Autodesk Fusion 360 part; units mm, degrees
(part 2 of 4)
  line L389 (379.0066, 108.4473) -> (374.6816, 115.9384)
  line L390 (374.6816, 115.9384) -> (377.3663, 117.4884)
  line L391 (377.3663, 117.4884) -> (381.6913, 109.9973)
  line L392 (383.1913, 109.9973) -> (394.9765, 130.4099)
  line L393 (394.2265, 131.7089) -> (385.5765, 131.7089)
  line L394 (385.5765, 131.7089) -> (385.5765, 134.8089)
  line L395 (385.5765, 134.8089) -> (394.2265, 134.8089)
  line L396 (394.9765, 136.1079) -> (383.1913, 156.5205)
  line L397 (381.6913, 156.5205) -> (377.3663, 149.0294)
  line L398 (377.3663, 149.0294) -> (374.6816, 150.5794)
  line L399 (374.6816, 150.5794) -> (379.0066, 158.0705)
  line L400 (378.2566, 159.3696) -> (354.6862, 159.3696)
  line L401 (353.9362, 158.0705) -> (358.2612, 150.5794)
  line L402 (358.2612, 150.5794) -> (355.5765, 149.0294)
  line L403 (355.5765, 149.0294) -> (351.2515, 156.5205)
  line L404 (349.7515, 156.5205) -> (337.9663, 136.1079)
  line L405 (338.7163, 134.8089) -> (347.3663, 134.8089)
  line L406 (347.3663, 134.8089) -> (347.3663, 131.7089)
  line L407 (347.3663, 131.7089) -> (338.7163, 131.7089)
  line L408 (254.1055, 108.9973) -> (242.3203, 129.4099)
  line L409 (240.8203, 129.4099) -> (236.4953, 121.9187)
  line L410 (236.4953, 121.9187) -> (233.8106, 123.4687)
  line L411 (233.8106, 123.4687) -> (238.1356, 130.9599)
  line L412 (237.3856, 132.2589) -> (213.8152, 132.2589)
  line L413 (213.0652, 130.9599) -> (217.3902, 123.4687)
  line L414 (217.3902, 123.4687) -> (214.7055, 121.9187)
  line L415 (214.7055, 121.9187) -> (210.3805, 129.4099)
  line L416 (208.8805, 129.4099) -> (197.0953, 108.9973)
  line L417 (197.8453, 107.6982) -> (206.4953, 107.6982)
  line L418 (206.4953, 107.6982) -> (206.4953, 104.5982)
  line L419 (206.4953, 104.5982) -> (197.8453, 104.5982)
  line L420 (197.0953, 103.2992) -> (208.8805, 82.8866)
  line L421 (210.3805, 82.8866) -> (214.7055, 90.3777)
  line L422 (214.7055, 90.3777) -> (217.3902, 88.8277)
  line L423 (217.3902, 88.8277) -> (213.0652, 81.3366)
  line L424 (213.8152, 80.0376) -> (237.3856, 80.0376)
  line L425 (238.1356, 81.3366) -> (233.8106, 88.8277)
  line L426 (233.8106, 88.8277) -> (236.4953, 90.3777)
  line L427 (236.4953, 90.3777) -> (240.8203, 82.8866)
  line L428 (242.3203, 82.8866) -> (254.1055, 103.2992)
  line L429 (253.3555, 104.5982) -> (244.7055, 104.5982)
  line L430 (244.7055, 104.5982) -> (244.7055, 107.6982)
  line L431 (244.7055, 107.6982) -> (253.3555, 107.6982)
  line L432 (337.9663, 184.6312) -> (349.7515, 164.2186)
  line L433 (351.2515, 164.2186) -> (355.5765, 171.7097)
  line L434 (355.5765, 171.7097) -> (358.2612, 170.1597)
  line L435 (358.2612, 170.1597) -> (353.9362, 162.6686)
  line L436 (354.6862, 161.3695) -> (378.2566, 161.3695)
  line L437 (379.0066, 162.6686) -> (374.6816, 170.1597)
  line L438 (374.6816, 170.1597) -> (377.3663, 171.7097)
  line L439 (377.3663, 171.7097) -> (381.6913, 164.2186)
  line L440 (383.1913, 164.2186) -> (394.9765, 184.6312)
  line L441 (394.2265, 185.9302) -> (385.5765, 185.9302)
  line L442 (385.5765, 185.9302) -> (385.5765, 189.0302)
  line L443 (385.5765, 189.0302) -> (394.2265, 189.0302)
  line L444 (394.9765, 190.3292) -> (383.1913, 210.7418)
  line L445 (381.6913, 210.7418) -> (377.3663, 203.2507)
  line L446 (377.3663, 203.2507) -> (374.6816, 204.8007)
  line L447 (374.6816, 204.8007) -> (379.0066, 212.2918)
  line L448 (378.2566, 213.5909) -> (354.6862, 213.5909)
  line L449 (353.9362, 212.2918) -> (358.2612, 204.8007)
  line L450 (358.2612, 204.8007) -> (355.5765, 203.2507)
  line L451 (355.5765, 203.2507) -> (351.2515, 210.7418)
  line L452 (349.7515, 210.7418) -> (337.9663, 190.3292)
  line L453 (338.7163, 189.0302) -> (347.3663, 189.0302)
  line L454 (347.3663, 189.0302) -> (347.3663, 185.9302)
  line L455 (347.3663, 185.9302) -> (338.7163, 185.9302)
  line L456 (244.0523, 238.8525) -> (255.8375, 218.4399)
  line L457 (257.3375, 218.4399) -> (261.6625, 225.931)
  line L458 (261.6625, 225.931) -> (264.3472, 224.381)
  line L459 (264.3472, 224.381) -> (260.0222, 216.8899)
  line L460 (260.7722, 215.5908) -> (284.3426, 215.5908)
  line L461 (285.0926, 216.8899) -> (280.7676, 224.381)
  line L462 (280.7676, 224.381) -> (283.4523, 225.931)
  line L463 (283.4523, 225.931) -> (287.7773, 218.4399)
  line L464 (289.2773, 218.4399) -> (301.0625, 238.8525)
  line L465 (300.3125, 240.1515) -> (291.6625, 240.1515)
  line L466 (291.6625, 240.1515) -> (291.6625, 243.2515)
  line L467 (291.6625, 243.2515) -> (300.3125, 243.2515)
  line L468 (301.0625, 244.5505) -> (289.2773, 264.9631)
  line L469 (287.7773, 264.9631) -> (283.4523, 257.472)
  line L470 (283.4523, 257.472) -> (280.7676, 259.022)
  line L471 (280.7676, 259.022) -> (285.0926, 266.5131)
  line L472 (284.3426, 267.8122) -> (260.7722, 267.8122)
  line L473 (260.0222, 266.5131) -> (264.3472, 259.022)
  line L474 (264.3472, 259.022) -> (261.6625, 257.472)
  line L475 (261.6625, 257.472) -> (257.3375, 264.9631)
  line L476 (255.8375, 264.9631) -> (244.0523, 244.5505)
  line L477 (244.8023, 243.2515) -> (253.4523, 243.2515)
  line L478 (253.4523, 243.2515) -> (253.4523, 240.1515)
  line L479 (253.4523, 240.1515) -> (244.8023, 240.1515)
  line L480 (291.0093, 49.0778) -> (302.7946, 28.6652)
  line L481 (304.2946, 28.6652) -> (308.6196, 36.1563)
  line L482 (308.6196, 36.1563) -> (311.3042, 34.6063)
  line L483 (311.3042, 34.6063) -> (306.9792, 27.1152)
  line L484 (307.7292, 25.8162) -> (331.2997, 25.8162)
  line L485 (332.0497, 27.1152) -> (327.7247, 34.6063)
  line L486 (327.7247, 34.6063) -> (330.4093, 36.1563)
  line L487 (330.4093, 36.1563) -> (334.7343, 28.6652)
  line L488 (336.2343, 28.6652) -> (348.0196, 49.0778)
  line L489 (347.2696, 50.3769) -> (338.6196, 50.3769)
  line L490 (338.6196, 50.3769) -> (338.6196, 53.4769)
  line L491 (338.6196, 53.4769) -> (347.2696, 53.4769)
  line L492 (348.0196, 54.7759) -> (336.2343, 75.1885)
  line L493 (334.7343, 75.1885) -> (330.4093, 67.6974)
  line L494 (330.4093, 67.6974) -> (327.7247, 69.2474)
  line L495 (327.7247, 69.2474) -> (332.0497, 76.7385)
  line L496 (331.2997, 78.0375) -> (307.7292, 78.0375)
  line L497 (306.9792, 76.7385) -> (311.3042, 69.2474)
  line L498 (311.3042, 69.2474) -> (308.6196, 67.6974)
  line L499 (308.6196, 67.6974) -> (304.2946, 75.1885)
  line L500 (302.7946, 75.1885) -> (291.0093, 54.7759)
  line L501 (291.7593, 53.4769) -> (300.4093, 53.4769)
  line L502 (300.4093, 53.4769) -> (300.4093, 50.3769)
  line L503 (300.4093, 50.3769) -> (291.7593, 50.3769)
  line L504 (291.0095, 374.4058) -> (302.7947, 353.9933)
  line L505 (304.2947, 353.9933) -> (308.6197, 361.4844)
  line L506 (308.6197, 361.4844) -> (311.3044, 359.9344)
  line L507 (311.3044, 359.9344) -> (306.9794, 352.4433)
  line L508 (307.7294, 351.1442) -> (331.2998, 351.1442)
  line L509 (332.0498, 352.4433) -> (327.7248, 359.9344)
  line L510 (327.7248, 359.9344) -> (330.4095, 361.4844)
  line L511 (330.4095, 361.4844) -> (334.7345, 353.9933)
  line L512 (336.2345, 353.9933) -> (348.0197, 374.4058)
  line L513 (347.2697, 375.7049) -> (338.6197, 375.7049)
  line L514 (338.6197, 375.7049) -> (338.6197, 378.8049)
  line L515 (338.6197, 378.8049) -> (347.2697, 378.8049)
  line L516 (348.0197, 380.1039) -> (336.2345, 400.5165)
  line L517 (334.7345, 400.5165) -> (330.4095, 393.0254)
  line L518 (330.4095, 393.0254) -> (327.7248, 394.5754)
  line L519 (327.7248, 394.5754) -> (332.0498, 402.0665)
  line L520 (331.2998, 403.3656) -> (307.7294, 403.3656)
  line L521 (306.9794, 402.0665) -> (311.3044, 394.5754)
  line L522 (311.3044, 394.5754) -> (308.6197, 393.0254)
  line L523 (308.6197, 393.0254) -> (304.2947, 400.5165)
  line L524 (302.7947, 400.5165) -> (291.0095, 380.1039)
  line L525 (291.7595, 378.8049) -> (300.4095, 378.8049)
  line L526 (300.4095, 378.8049) -> (300.4095, 375.7049)
  line L527 (300.4095, 375.7049) -> (291.7595, 375.7049)
  line L528 (301.0626, 136.1079) -> (289.2774, 156.5205)
  line L529 (287.7774, 156.5205) -> (283.4524, 149.0294)
  line L530 (283.4524, 149.0294) -> (280.7677, 150.5794)
  line L531 (280.7677, 150.5794) -> (285.0927, 158.0705)
  line L532 (284.3427, 159.3695) -> (260.7722, 159.3695)
  line L533 (260.0222, 158.0705) -> (264.3472, 150.5794)
  line L534 (264.3472, 150.5794) -> (261.6626, 149.0294)
  line L535 (261.6626, 149.0294) -> (257.3376, 156.5205)
  line L536 (255.8376, 156.5205) -> (244.0524, 136.1079)
  line L537 (244.8024, 134.8088) -> (253.4524, 134.8088)
  line L538 (253.4524, 134.8088) -> (253.4524, 131.7088)
  line L539 (253.4524, 131.7088) -> (244.8024, 131.7088)
  line L540 (244.0524, 130.4098) -> (255.8376, 109.9972)
  line L541 (257.3376, 109.9972) -> (261.6626, 117.4883)
  line L542 (261.6626, 117.4883) -> (264.3472, 115.9383)
  line L543 (264.3472, 115.9383) -> (260.0222, 108.4472)
  line L544 (260.7722, 107.1482) -> (284.3427, 107.1482)
  line L545 (285.0927, 108.4472) -> (280.7677, 115.9383)
  line L546 (280.7677, 115.9383) -> (283.4524, 117.4883)
  line L547 (283.4524, 117.4883) -> (287.7774, 109.9972)
  line L548 (289.2774, 109.9972) -> (301.0626, 130.4098)
  line L549 (300.3126, 131.7088) -> (291.6626, 131.7088)
  line L550 (291.6626, 131.7088) -> (291.6626, 134.8088)
  line L551 (291.6626, 134.8088) -> (300.3126, 134.8088)
  line L552 (291.0093, 320.1845) -> (302.7945, 299.7719)
  line L553 (304.2945, 299.7719) -> (308.6195, 307.263)
  line L554 (308.6195, 307.263) -> (311.3042, 305.713)
  line L555 (311.3042, 305.713) -> (306.9792, 298.2219)
  line L556 (307.7292, 296.9229) -> (331.2996, 296.9229)
  line L557 (332.0496, 298.2219) -> (327.7246, 305.713)
  line L558 (327.7246, 305.713) -> (330.4093, 307.263)
  line L559 (330.4093, 307.263) -> (334.7343, 299.7719)
  line L560 (336.2343, 299.7719) -> (348.0195, 320.1845)
  line L561 (347.2695, 321.4836) -> (338.6195, 321.4836)
  line L562 (338.6195, 321.4836) -> (338.6195, 324.5836)
  line L563 (338.6195, 324.5836) -> (347.2695, 324.5836)
  line L564 (348.0195, 325.8826) -> (336.2343, 346.2952)
  line L565 (334.7343, 346.2952) -> (330.4093, 338.8041)
  line L566 (330.4093, 338.8041) -> (327.7246, 340.3541)
  line L567 (327.7246, 340.3541) -> (332.0496, 347.8452)
  line L568 (331.2996, 349.1442) -> (307.7292, 349.1442)
  line L569 (306.9792, 347.8452) -> (311.3042, 340.3541)
  line L570 (311.3042, 340.3541) -> (308.6195, 338.8041)
  line L571 (308.6195, 338.8041) -> (304.2945, 346.2952)
  line L572 (302.7945, 346.2952) -> (291.0093, 325.8826)
  line L573 (291.7593, 324.5836) -> (300.4093, 324.5836)
  line L574 (300.4093, 324.5836) -> (300.4093, 321.4836)
  line L575 (300.4093, 321.4836) -> (291.7593, 321.4836)
  line L576 (384.9234, 320.1844) -> (396.7086, 299.7719)
  line L577 (398.2086, 299.7719) -> (402.5336, 307.263)
  line L578 (402.5336, 307.263) -> (405.2183, 305.713)
  line L579 (405.2183, 305.713) -> (400.8933, 298.2219)
  line L580 (401.6433, 296.9228) -> (425.2137, 296.9228)
  line L581 (425.9637, 298.2219) -> (421.6387, 305.713)
  line L582 (421.6387, 305.713) -> (424.3234, 307.263)
  line L583 (424.3234, 307.263) -> (428.6484, 299.7719)
  line L584 (430.1484, 299.7719) -> (441.9336, 320.1844)
  line L585 (441.1836, 321.4835) -> (432.5336, 321.4835)
  line L586 (432.5336, 321.4835) -> (432.5336, 324.5835)
  line L587 (432.5336, 324.5835) -> (441.1836, 324.5835)
  line L588 (441.9336, 325.8825) -> (430.1484, 346.2951)
  line L589 (428.6484, 346.2951) -> (424.3234, 338.804)
  line L590 (424.3234, 338.804) -> (421.6387, 340.354)
  line L591 (421.6387, 340.354) -> (425.9637, 347.8451)
  line L592 (425.2137, 349.1441) -> (401.6433, 349.1441)
  line L593 (400.8933, 347.8451) -> (405.2183, 340.354)
  line L594 (405.2183, 340.354) -> (402.5336, 338.804)
  line L595 (402.5336, 338.804) -> (398.2086, 346.2951)
  line L596 (396.7086, 346.2951) -> (384.9234, 325.8825)
  line L597 (385.6734, 324.5835) -> (394.3234, 324.5835)
  line L598 (394.3234, 324.5835) -> (394.3234, 321.4835)
  line L599 (394.3234, 321.4835) -> (385.6734, 321.4835)
  line L600 (291.0093, 103.2992) -> (302.7946, 82.8866)
  line L601 (304.2946, 82.8866) -> (308.6196, 90.3777)
  line L602 (308.6196, 90.3777) -> (311.3042, 88.8277)
  line L603 (311.3042, 88.8277) -> (306.9792, 81.3366)
  line L604 (307.7292, 80.0376) -> (331.2997, 80.0376)
  line L605 (332.0497, 81.3366) -> (327.7247, 88.8277)
  line L606 (327.7247, 88.8277) -> (330.4093, 90.3777)
  line L607 (330.4093, 90.3777) -> (334.7343, 82.8866)
  line L608 (336.2343, 82.8866) -> (348.0196, 103.2992)
  line L609 (347.2696, 104.5982) -> (338.6196, 104.5982)
  line L610 (338.6196, 104.5982) -> (338.6196, 107.6982)
  line L611 (338.6196, 107.6982) -> (347.2696, 107.6982)
  line L612 (348.0196, 108.9973) -> (336.2343, 129.4099)
  line L613 (334.7343, 129.4099) -> (330.4093, 121.9187)
  line L614 (330.4093, 121.9187) -> (327.7247, 123.4687)
  line L615 (327.7247, 123.4687) -> (332.0497, 130.9599)
  line L616 (331.2997, 132.2589) -> (307.7292, 132.2589)
  line L617 (306.9792, 130.9599) -> (311.3042, 123.4687)
  line L618 (311.3042, 123.4687) -> (308.6196, 121.9187)
  line L619 (308.6196, 121.9187) -> (304.2946, 129.4099)
  line L620 (302.7946, 129.4099) -> (291.0093, 108.9973)
  line L621 (291.7593, 107.6982) -> (300.4093, 107.6982)
  line L622 (300.4093, 107.6982) -> (300.4093, 104.5982)
  line L623 (300.4093, 104.5982) -> (291.7593, 104.5982)
  line L624 (291.0093, 265.9632) -> (302.7945, 245.5506)
  line L625 (304.2945, 245.5506) -> (308.6195, 253.0417)
  line L626 (308.6195, 253.0417) -> (311.3042, 251.4917)
  line L627 (311.3042, 251.4917) -> (306.9792, 244.0006)
  line L628 (307.7292, 242.7015) -> (331.2996, 242.7015)
  line L629 (332.0496, 244.0006) -> (327.7246, 251.4917)
  line L630 (327.7246, 251.4917) -> (330.4093, 253.0417)
  line L631 (330.4093, 253.0417) -> (334.7343, 245.5506)
  line L632 (336.2343, 245.5506) -> (348.0195, 265.9632)
  line L633 (347.2695, 267.2622) -> (338.6195, 267.2622)
  line L634 (338.6195, 267.2622) -> (338.6195, 270.3622)
  line L635 (338.6195, 270.3622) -> (347.2695, 270.3622)
  line L636 (348.0195, 271.6612) -> (336.2343, 292.0738)
  line L637 (334.7343, 292.0738) -> (330.4093, 284.5827)
  line L638 (330.4093, 284.5827) -> (327.7246, 286.1327)
  line L639 (327.7246, 286.1327) -> (332.0496, 293.6238)
  line L640 (331.2996, 294.9229) -> (307.7292, 294.9229)
  line L641 (306.9792, 293.6238) -> (311.3042, 286.1327)
  line L642 (311.3042, 286.1327) -> (308.6195, 284.5827)
  line L643 (308.6195, 284.5827) -> (304.2945, 292.0738)
  line L644 (302.7945, 292.0738) -> (291.0093, 271.6612)
  line L645 (291.7593, 270.3622) -> (300.4093, 270.3622)
  line L646 (300.4093, 270.3622) -> (300.4093, 267.2622)
  line L647 (300.4093, 267.2622) -> (291.7593, 267.2622)
  line L648 (337.9664, 238.8525) -> (349.7516, 218.4399)
  line L649 (351.2516, 218.4399) -> (355.5766, 225.931)
  line L650 (355.5766, 225.931) -> (358.2613, 224.381)
  line L651 (358.2613, 224.381) -> (353.9363, 216.8899)
  line L652 (354.6863, 215.5909) -> (378.2567, 215.5909)
  line L653 (379.0067, 216.8899) -> (374.6817, 224.381)
  line L654 (374.6817, 224.381) -> (377.3664, 225.931)
  line L655 (377.3664, 225.931) -> (381.6914, 218.4399)
  line L656 (383.1914, 218.4399) -> (394.9766, 238.8525)
  line L657 (394.2266, 240.1515) -> (385.5766, 240.1515)
  line L658 (385.5766, 240.1515) -> (385.5766, 243.2515)
  line L659 (385.5766, 243.2515) -> (394.2266, 243.2515)
  line L660 (394.9766, 244.5506) -> (383.1914, 264.9632)
  line L661 (381.6914, 264.9632) -> (377.3664, 257.472)
  line L662 (377.3664, 257.472) -> (374.6817, 259.022)
  line L663 (374.6817, 259.022) -> (379.0067, 266.5132)
  line L664 (378.2567, 267.8122) -> (354.6863, 267.8122)
  line L665 (353.9363, 266.5132) -> (358.2613, 259.022)
  line L666 (358.2613, 259.022) -> (355.5766, 257.472)
  line L667 (355.5766, 257.472) -> (351.2516, 264.9632)
  line L668 (349.7516, 264.9632) -> (337.9664, 244.5506)
  line L669 (338.7164, 243.2515) -> (347.3664, 243.2515)
  line L670 (347.3664, 243.2515) -> (347.3664, 240.1515)
  line L671 (347.3664, 240.1515) -> (338.7164, 240.1515)
  line L672 (384.9234, 103.2992) -> (396.7086, 82.8866)
  line L673 (398.2086, 82.8866) -> (402.5336, 90.3777)
  line L674 (402.5336, 90.3777) -> (405.2183, 88.8277)
  line L675 (405.2183, 88.8277) -> (400.8933, 81.3366)
  line L676 (401.6433, 80.0376) -> (425.2137, 80.0376)
  line L677 (425.9637, 81.3366) -> (421.6387, 88.8277)
  line L678 (421.6387, 88.8277) -> (424.3234, 90.3777)
  line L679 (424.3234, 90.3777) -> (428.6484, 82.8866)
  line L680 (430.1484, 82.8866) -> (441.9336, 103.2992)
  line L681 (441.1836, 104.5982) -> (432.5336, 104.5982)
  line L682 (432.5336, 104.5982) -> (432.5336, 107.6982)
  line L683 (432.5336, 107.6982) -> (441.1836, 107.6982)
  line L684 (441.9336, 108.9973) -> (430.1484, 129.4099)
  line L685 (428.6484, 129.4099) -> (424.3234, 121.9187)
  line L686 (424.3234, 121.9187) -> (421.6387, 123.4687)
  line L687 (421.6387, 123.4687) -> (425.9637, 130.9599)
  line L688 (425.2137, 132.2589) -> (401.6433, 132.2589)
  line L689 (400.8933, 130.9599) -> (405.2183, 123.4687)
  line L690 (405.2183, 123.4687) -> (402.5336, 121.9187)
  line L691 (402.5336, 121.9187) -> (398.2086, 129.4099)
  line L692 (396.7086, 129.4099) -> (384.9234, 108.9973)
  line L693 (385.6734, 107.6982) -> (394.3234, 107.6982)
  line L694 (394.3234, 107.6982) -> (394.3234, 104.5982)
  line L695 (394.3234, 104.5982) -> (385.6734, 104.5982)
  line L696 (384.9234, 211.7419) -> (396.7086, 191.3293)
  line L697 (398.2086, 191.3293) -> (402.5336, 198.8204)
  line L698 (402.5336, 198.8204) -> (405.2183, 197.2704)
  line L699 (405.2183, 197.2704) -> (400.8933, 189.7793)
  line L700 (401.6433, 188.4802) -> (425.2137, 188.4802)
  line L701 (425.9637, 189.7793) -> (421.6387, 197.2704)
  line L702 (421.6387, 197.2704) -> (424.3234, 198.8204)
  line L703 (424.3234, 198.8204) -> (428.6484, 191.3293)
  line L704 (430.1484, 191.3293) -> (441.9336, 211.7419)
  line L705 (441.1836, 213.0409) -> (432.5336, 213.0409)
  line L706 (432.5336, 213.0409) -> (432.5336, 216.1409)
  line L707 (432.5336, 216.1409) -> (441.1836, 216.1409)
  line L708 (441.9336, 217.44) -> (430.1484, 237.8525)
  line L709 (428.6484, 237.8525) -> (424.3234, 230.3614)
  line L710 (424.3234, 230.3614) -> (421.6387, 231.9114)
  line L711 (421.6387, 231.9114) -> (425.9637, 239.4025)
  line L712 (425.2137, 240.7016) -> (401.6433, 240.7016)
  line L713 (400.8933, 239.4025) -> (405.2183, 231.9114)
  line L714 (405.2183, 231.9114) -> (402.5336, 230.3614)
  line L715 (402.5336, 230.3614) -> (398.2086, 237.8525)
  line L716 (396.7086, 237.8525) -> (384.9234, 217.44)
  line L717 (385.6734, 216.1409) -> (394.3234, 216.1409)
  line L718 (394.3234, 216.1409) -> (394.3234, 213.0409)
  line L719 (394.3234, 213.0409) -> (385.6734, 213.0409)
  line L720 (384.9234, 49.0778) -> (396.7086, 28.6652)
  line L721 (398.2086, 28.6652) -> (402.5336, 36.1563)
  line L722 (402.5336, 36.1563) -> (405.2183, 34.6063)
  line L723 (405.2183, 34.6063) -> (400.8933, 27.1152)
  line L724 (401.6433, 25.8162) -> (425.2137, 25.8162)
  line L725 (425.9637, 27.1152) -> (421.6387, 34.6063)
  line L726 (421.6387, 34.6063) -> (424.3234, 36.1563)
  line L727 (424.3234, 36.1563) -> (428.6484, 28.6652)
  line L728 (430.1484, 28.6652) -> (441.9336, 49.0778)
  line L729 (441.1836, 50.3769) -> (432.5336, 50.3769)
  line L730 (432.5336, 50.3769) -> (432.5336, 53.4769)
  line L731 (432.5336, 53.4769) -> (441.1836, 53.4769)
  line L732 (441.9336, 54.7759) -> (430.1484, 75.1885)
  line L733 (428.6484, 75.1885) -> (424.3234, 67.6974)
  line L734 (424.3234, 67.6974) -> (421.6387, 69.2474)
  line L735 (421.6387, 69.2474) -> (425.9637, 76.7385)
  line L736 (425.2137, 78.0375) -> (401.6433, 78.0375)
  line L737 (400.8933, 76.7385) -> (405.2183, 69.2474)
  line L738 (405.2183, 69.2474) -> (402.5336, 67.6974)
  line L739 (402.5336, 67.6974) -> (398.2086, 75.1885)
  line L740 (396.7086, 75.1885) -> (384.9234, 54.7759)
  line L741 (385.6734, 53.4769) -> (394.3234, 53.4769)
  line L742 (394.3234, 53.4769) -> (394.3234, 50.3769)
  line L743 (394.3234, 50.3769) -> (385.6734, 50.3769)
  line L744 (301.0628, 190.3292) -> (289.2776, 210.7418)
  line L745 (287.7776, 210.7418) -> (283.4526, 203.2507)
  line L746 (283.4526, 203.2507) -> (280.7679, 204.8007)
  line L747 (280.7679, 204.8007) -> (285.0929, 212.2918)
  line L748 (284.3429, 213.5908) -> (260.7725, 213.5908)
  line L749 (260.0225, 212.2918) -> (264.3475, 204.8007)
  line L750 (264.3475, 204.8007) -> (261.6628, 203.2507)
  line L751 (261.6628, 203.2507) -> (257.3378, 210.7418)
  line L752 (255.8378, 210.7418) -> (244.0526, 190.3292)
  line L753 (244.8026, 189.0302) -> (253.4526, 189.0302)
  line L754 (253.4526, 189.0302) -> (253.4526, 185.9302)
  line L755 (253.4526, 185.9302) -> (244.8026, 185.9302)
  line L756 (244.0526, 184.6311) -> (255.8378, 164.2185)
  line L757 (257.3378, 164.2185) -> (261.6628, 171.7097)
  line L758 (261.6628, 171.7097) -> (264.3475, 170.1597)
  line L759 (264.3475, 170.1597) -> (260.0225, 162.6685)
  line L760 (260.7725, 161.3695) -> (284.3429, 161.3695)
  line L761 (285.0929, 162.6685) -> (280.7679, 170.1597)
  line L762 (280.7679, 170.1597) -> (283.4526, 171.7097)
  line L763 (283.4526, 171.7097) -> (287.7776, 164.2185)
  line L764 (289.2776, 164.2185) -> (301.0628, 184.6311)
  line L765 (300.3128, 185.9302) -> (291.6628, 185.9302)
  line L766 (291.6628, 185.9302) -> (291.6628, 189.0302)
  line L767 (291.6628, 189.0302) -> (300.3128, 189.0302)
  line L768 (337.9663, 76.1885) -> (349.7515, 55.7759)
  line L769 (351.2515, 55.7759) -> (355.5765, 63.267)
  line L770 (355.5765, 63.267) -> (358.2612, 61.717)
  line L771 (358.2612, 61.717) -> (353.9362, 54.2259)
  line L772 (354.6862, 52.9269) -> (378.2566, 52.9269)
  line L773 (379.0066, 54.2259) -> (374.6816, 61.717)
  line L774 (374.6816, 61.717) -> (377.3663, 63.267)
  line L775 (377.3663, 63.267) -> (381.6913, 55.7759)
  line L776 (383.1913, 55.7759) -> (394.9765, 76.1885)
  line L777 (394.2265, 77.4875) -> (385.5765, 77.4875)
  line L778 (385.5765, 77.4875) -> (385.5765, 80.5875)
  line L779 (385.5765, 80.5875) -> (394.2265, 80.5875)
  line L780 (394.9765, 81.8866) -> (383.1913, 102.2992)
  line L781 (381.6913, 102.2992) -> (377.3663, 94.808)
  line L782 (377.3663, 94.808) -> (374.6816, 96.358)
  line L783 (374.6816, 96.358) -> (379.0066, 103.8492)
  line L784 (378.2566, 105.1482) -> (354.6862, 105.1482)
  line L785 (353.9362, 103.8492) -> (358.2612, 96.358)
  line L786 (358.2612, 96.358) -> (355.5765, 94.808)
  line L787 (355.5765, 94.808) -> (351.2515, 102.2992)
  line L788 (349.7515, 102.2992) -> (337.9663, 81.8866)
  line L789 (338.7163, 80.5875) -> (347.3663, 80.5875)
  line L790 (347.3663, 80.5875) -> (347.3663, 77.4875)
  line L791 (347.3663, 77.4875) -> (338.7163, 77.4875)
  line L792 (301.0626, 81.8866) -> (289.2774, 102.2992)
  line L793 (287.7774, 102.2992) -> (283.4524, 94.8081)
  line L794 (283.4524, 94.8081) -> (280.7677, 96.3581)
  line L795 (280.7677, 96.3581) -> (285.0927, 103.8492)
  line L796 (284.3427, 105.1482) -> (260.7722, 105.1482)
  line L797 (260.0222, 103.8492) -> (264.3472, 96.3581)
  line L798 (264.3472, 96.3581) -> (261.6626, 94.8081)
  line L799 (261.6626, 94.8081) -> (257.3376, 102.2992)
  line L800 (255.8376, 102.2992) -> (244.0524, 81.8866)
  line L801 (244.8024, 80.5876) -> (253.4524, 80.5876)
  line L802 (253.4524, 80.5876) -> (253.4524, 77.4876)
  line L803 (253.4524, 77.4876) -> (244.8024, 77.4876)
  line L804 (244.0524, 76.1885) -> (255.8376, 55.7759)
  line L805 (257.3376, 55.7759) -> (261.6626, 63.267)
  line L806 (261.6626, 63.267) -> (264.3472, 61.717)
  line L807 (264.3472, 61.717) -> (260.0222, 54.2259)
  line L808 (260.7722, 52.9269) -> (284.3427, 52.9269)
  line L809 (285.0927, 54.2259) -> (280.7677, 61.717)
  line L810 (280.7677, 61.717) -> (283.4524, 63.267)
  line L811 (283.4524, 63.267) -> (287.7774, 55.7759)
  line L812 (289.2774, 55.7759) -> (301.0626, 76.1885)
  line L813 (300.3126, 77.4876) -> (291.6626, 77.4876)
  line L814 (291.6626, 77.4876) -> (291.6626, 80.5876)
  line L815 (291.6626, 80.5876) -> (300.3126, 80.5876)
  line L816 (384.9234, 157.5205) -> (396.7086, 137.1079)
  line L817 (398.2086, 137.1079) -> (402.5336, 144.5991)
  line L818 (402.5336, 144.5991) -> (405.2183, 143.0491)
  line L819 (405.2183, 143.0491) -> (400.8933, 135.5579)
  line L820 (401.6433, 134.2589) -> (425.2137, 134.2589)
  line L821 (425.9637, 135.5579) -> (421.6387, 143.0491)
  line L822 (421.6387, 143.0491) -> (424.3234, 144.5991)
  line L823 (424.3234, 144.5991) -> (428.6484, 137.1079)
  line L824 (430.1484, 137.1079) -> (441.9336, 157.5205)
  line L825 (441.1836, 158.8196) -> (432.5336, 158.8196)
  line L826 (432.5336, 158.8196) -> (432.5336, 161.9196)
  line L827 (432.5336, 161.9196) -> (441.1836, 161.9196)
  line L828 (441.9336, 163.2186) -> (430.1484, 183.6312)
  line L829 (428.6484, 183.6312) -> (424.3234, 176.1401)
  line L830 (424.3234, 176.1401) -> (421.6387, 177.6901)
  line L831 (421.6387, 177.6901) -> (425.9637, 185.1812)
  line L832 (425.2137, 186.4802) -> (401.6433, 186.4802)
  line L833 (400.8933, 185.1812) -> (405.2183, 177.6901)
  line L834 (405.2183, 177.6901) -> (402.5336, 176.1401)
  line L835 (402.5336, 176.1401) -> (398.2086, 183.6312)
  line L836 (396.7086, 183.6312) -> (384.9234, 163.2186)
  line L837 (385.6734, 161.9196) -> (394.3234, 161.9196)
  line L838 (394.3234, 161.9196) -> (394.3234, 158.8196)
  line L839 (394.3234, 158.8196) -> (385.6734, 158.8196)
  line L840 (384.9234, 265.9632) -> (396.7086, 245.5506)
  line L841 (398.2086, 245.5506) -> (402.5336, 253.0417)
  line L842 (402.5336, 253.0417) -> (405.2183, 251.4917)
  line L843 (405.2183, 251.4917) -> (400.8933, 244.0006)
  line L844 (401.6433, 242.7016) -> (425.2137, 242.7016)
  line L845 (425.9637, 244.0006) -> (421.6387, 251.4917)
  line L846 (421.6387, 251.4917) -> (424.3234, 253.0417)
  line L847 (424.3234, 253.0417) -> (428.6484, 245.5506)
  line L848 (430.1484, 245.5506) -> (441.9336, 265.9632)
  line L849 (441.1836, 267.2622) -> (432.5336, 267.2622)
  line L850 (432.5336, 267.2622) -> (432.5336, 270.3622)
  line L851 (432.5336, 270.3622) -> (441.1836, 270.3622)
  line L852 (441.9336, 271.6613) -> (430.1484, 292.0739)
  line L853 (428.6484, 292.0739) -> (424.3234, 284.5827)
  line L854 (424.3234, 284.5827) -> (421.6387, 286.1327)
  line L855 (421.6387, 286.1327) -> (425.9637, 293.6239)
  line L856 (425.2137, 294.9229) -> (401.6433, 294.9229)
  line L857 (400.8933, 293.6239) -> (405.2183, 286.1327)
  line L858 (405.2183, 286.1327) -> (402.5336, 284.5827)
  line L859 (402.5336, 284.5827) -> (398.2086, 292.0739)
  line L860 (396.7086, 292.0739) -> (384.9234, 271.6613)
  line L861 (385.6734, 270.3622) -> (394.3234, 270.3622)
  line L862 (394.3234, 270.3622) -> (394.3234, 267.2622)
  line L863 (394.3234, 267.2622) -> (385.6734, 267.2622)
  line L864 (35.4525, 215.6624) -> (35.4525, 193.6374)
  line L865 (36.9525, 192.1374) -> (45.6025, 192.1374)
  line L866 (45.6025, 192.1374) -> (45.6025, 189.0374)
  line L867 (45.6025, 189.0374) -> (36.9525, 189.0374)
  line L868 (35.4525, 187.5374) -> (35.4525, 165.5124)
  line L869 (35.4525, 165.5124) -> (57.4775, 165.5124)
  line L870 (58.9775, 167.0124) -> (58.9775, 175.6624)
  line L871 (58.9775, 175.6624) -> (62.0775, 175.6624)
  line L872 (62.0775, 175.6624) -> (62.0775, 167.0124)
  line L873 (63.5775, 165.5124) -> (85.6025, 165.5124)
  line L874 (85.6025, 165.5124) -> (85.6025, 187.5374)
  line L875 (84.1025, 189.0374) -> (75.4525, 189.0374)
  line L876 (75.4525, 189.0374) -> (75.4525, 192.1374)
  line L877 (75.4525, 192.1374) -> (84.1025, 192.1374)
  line L878 (85.6025, 193.6374) -> (85.6025, 215.6624)
  line L879 (85.6025, 215.6624) -> (63.5775, 215.6624)
  line L880 (62.0775, 214.1624) -> (62.0775, 205.5124)
  line L881 (62.0775, 205.5124) -> (58.9775, 205.5124)
  line L882 (58.9775, 205.5124) -> (58.9775, 214.1624)
  line L883 (57.4775, 215.6624) -> (35.4525, 215.6624)
  line L884 (82.4091, 372.1123) -> (82.4091, 350.0873)
  line L885 (83.9091, 348.5873) -> (92.5591, 348.5873)
  line L886 (92.5591, 348.5873) -> (92.5591, 345.4873)
  line L887 (92.5591, 345.4873) -> (83.9091, 345.4873)
  line L888 (82.4091, 343.9873) -> (82.4091, 321.9623)
  line L889 (82.4091, 321.9623) -> (104.4341, 321.9623)
  line L890 (105.9341, 323.4623) -> (105.9341, 332.1123)
  line L891 (105.9341, 332.1123) -> (109.0341, 332.1123)
  line L892 (109.0341, 332.1123) -> (109.0341, 323.4623)
  line L893 (110.5341, 321.9623) -> (132.5591, 321.9623)
  line L894 (132.5591, 321.9623) -> (132.5591, 343.9873)
  line L895 (131.0591, 345.4873) -> (122.4091, 345.4873)
  line L896 (122.4091, 345.4873) -> (122.4091, 348.5873)
  line L897 (122.4091, 348.5873) -> (131.0591, 348.5873)
  line L898 (132.5591, 350.0873) -> (132.5591, 372.1123)
  line L899 (132.5591, 372.1123) -> (110.5341, 372.1123)
  line L900 (109.0341, 370.6123) -> (109.0341, 361.9623)
  line L901 (109.0341, 361.9623) -> (105.9341, 361.9623)
  line L902 (105.9341, 361.9623) -> (105.9341, 370.6123)
  line L903 (104.4341, 372.1123) -> (82.4091, 372.1123)
  line L904 (144.9454, 128.1162) -> (144.9454, 106.0912)
  line L905 (146.4454, 104.5912) -> (155.0954, 104.5912)
  line L906 (155.0954, 104.5912) -> (155.0954, 101.4912)
  line L907 (155.0954, 101.4912) -> (146.4454, 101.4912)
  line L908 (144.9454, 99.9912) -> (144.9454, 77.9662)
  line L909 (144.9454, 77.9662) -> (166.9704, 77.9662)
  line L910 (168.4704, 79.4662) -> (168.4704, 88.1162)
  line L911 (168.4704, 88.1162) -> (171.5704, 88.1162)
  line L912 (171.5704, 88.1162) -> (171.5704, 79.4662)
  line L913 (173.0704, 77.9662) -> (195.0954, 77.9662)
  line L914 (195.0954, 77.9662) -> (195.0954, 99.9912)
  line L915 (193.5954, 101.4912) -> (184.9454, 101.4912)
  line L916 (184.9454, 101.4912) -> (184.9454, 104.5912)
  line L917 (184.9454, 104.5912) -> (193.5954, 104.5912)
  line L918 (195.0954, 106.0912) -> (195.0954, 128.1162)
  line L919 (195.0954, 128.1162) -> (173.0704, 128.1162)
  line L920 (171.5704, 126.6162) -> (171.5704, 117.9662)
  line L921 (171.5704, 117.9662) -> (168.4704, 117.9662)
  line L922 (168.4704, 117.9662) -> (168.4704, 126.6162)
  line L923 (166.9704, 128.1162) -> (144.9454, 128.1162)
  line L924 (139.7525, 215.6621) -> (139.7525, 193.6371)
  line L925 (141.2525, 192.1371) -> (149.9025, 192.1371)
  line L926 (149.9025, 192.1371) -> (149.9025, 189.0371)
  line L927 (149.9025, 189.0371) -> (141.2525, 189.0371)
  line L928 (139.7525, 187.5371) -> (139.7525, 165.5121)
  line L929 (139.7525, 165.5121) -> (161.7775, 165.5121)
  line L930 (163.2775, 167.0121) -> (163.2775, 175.6621)
  line L931 (163.2775, 175.6621) -> (166.3775, 175.6621)
  line L932 (166.3775, 175.6621) -> (166.3775, 167.0121)
  line L933 (167.8775, 165.5121) -> (189.9025, 165.5121)
  line L934 (189.9025, 165.5121) -> (189.9025, 187.5371)
  line L935 (188.4025, 189.0371) -> (179.7525, 189.0371)
  line L936 (179.7525, 189.0371) -> (179.7525, 192.1371)
  line L937 (179.7525, 192.1371) -> (188.4025, 192.1371)
  line L938 (189.9025, 193.6371) -> (189.9025, 215.6621)
  line L939 (189.9025, 215.6621) -> (167.8775, 215.6621)
  line L940 (166.3775, 214.1621) -> (166.3775, 205.5121)
  line L941 (166.3775, 205.5121) -> (163.2775, 205.5121)
  line L942 (163.2775, 205.5121) -> (163.2775, 214.1621)
  line L943 (161.7775, 215.6621) -> (139.7525, 215.6621)
  line L944 (238.8593, 319.9622) -> (238.8593, 297.9372)
  line L945 (240.3593, 296.4372) -> (249.0093, 296.4372)
  line L946 (249.0093, 296.4372) -> (249.0093, 293.3372)
  line L947 (249.0093, 293.3372) -> (240.3593, 293.3372)
  line L948 (238.8593, 291.8372) -> (238.8593, 269.8122)
  line L949 (238.8593, 269.8122) -> (260.8843, 269.8122)
  line L950 (262.3843, 271.3122) -> (262.3843, 279.9622)
  line L951 (262.3843, 279.9622) -> (265.4843, 279.9622)
  line L952 (265.4843, 279.9622) -> (265.4843, 271.3122)
  line L953 (266.9843, 269.8122) -> (289.0093, 269.8122)
  line L954 (289.0093, 269.8122) -> (289.0093, 291.8372)
  line L955 (287.5093, 293.3372) -> (278.8593, 293.3372)
  line L956 (278.8593, 293.3372) -> (278.8593, 296.4372)
  line L957 (278.8593, 296.4372) -> (287.5093, 296.4372)
  line L958 (289.0093, 297.9372) -> (289.0093, 319.9622)
  line L959 (289.0093, 319.9622) -> (266.9843, 319.9622)
  line L960 (265.4843, 318.4622) -> (265.4843, 309.8122)
  line L961 (265.4843, 309.8122) -> (262.3843, 309.8122)
  line L962 (262.3843, 309.8122) -> (262.3843, 318.4622)
  line L963 (260.8843, 319.9622) -> (238.8593, 319.9622)
  line L964 (238.8594, 372.1122) -> (238.8594, 350.0872)
  line L965 (240.3594, 348.5872) -> (249.0094, 348.5872)
  line L966 (249.0094, 348.5872) -> (249.0094, 345.4872)
  line L967 (249.0094, 345.4872) -> (240.3594, 345.4872)
  line L968 (238.8594, 343.9872) -> (238.8594, 321.9622)
  line L969 (238.8594, 321.9622) -> (260.8844, 321.9622)
  line L970 (262.3844, 323.4622) -> (262.3844, 332.1122)
  line L971 (262.3844, 332.1122) -> (265.4844, 332.1122)
  line L972 (265.4844, 332.1122) -> (265.4844, 323.4622)
  line L973 (266.9844, 321.9622) -> (289.0094, 321.9622)
  line L974 (289.0094, 321.9622) -> (289.0094, 343.9872)
  line L975 (287.5094, 345.4872) -> (278.8594, 345.4872)
  line L976 (278.8594, 345.4872) -> (278.8594, 348.5872)
  line L977 (278.8594, 348.5872) -> (287.5094, 348.5872)
  line L978 (289.0094, 350.0872) -> (289.0094, 372.1122)
  line L979 (289.0094, 372.1122) -> (266.9844, 372.1122)
  line L980 (265.4844, 370.6122) -> (265.4844, 361.9622)
  line L981 (265.4844, 361.9622) -> (262.3844, 361.9622)
  line L982 (262.3844, 361.9622) -> (262.3844, 370.6122)
  line L983 (260.8844, 372.1122) -> (238.8594, 372.1122)
  line L984 (189.9026, 217.6621) -> (189.9026, 239.6871)
  line L985 (188.4026, 241.1871) -> (179.7526, 241.1871)
  line L986 (179.7526, 241.1871) -> (179.7526, 244.2871)
  line L987 (179.7526, 244.2871) -> (188.4026, 244.2871)
  line L988 (189.9026, 245.7871) -> (189.9026, 267.8121)
  line L989 (189.9026, 267.8121) -> (167.8776, 267.8121)
  line L990 (166.3776, 266.3121) -> (166.3776, 257.6621)
  line L991 (166.3776, 257.6621) -> (163.2776, 257.6621)
  line L992 (163.2776, 257.6621) -> (163.2776, 266.3121)
  line L993 (161.7776, 267.8121) -> (139.7526, 267.8121)
  line L994 (139.7526, 267.8121) -> (139.7526, 245.7871)
  line L995 (141.2526, 244.2871) -> (149.9026, 244.2871)
  line L996 (149.9026, 244.2871) -> (149.9026, 241.1871)
  line L997 (149.9026, 241.1871) -> (141.2526, 241.1871)
  line L998 (139.7526, 239.6871) -> (139.7526, 217.6621)
  line L999 (139.7526, 217.6621) -> (161.7776, 217.6621)
  line L1000 (163.2776, 219.1621) -> (163.2776, 227.8121)
  line L1001 (163.2776, 227.8121) -> (166.3776, 227.8121)
  line L1002 (166.3776, 227.8121) -> (166.3776, 219.1621)
  line L1003 (167.8776, 217.6621) -> (189.9026, 217.6621)
  line L1004 (90.7952, 75.9662) -> (68.7702, 75.9662)
  line L1005 (67.2702, 74.4662) -> (67.2702, 65.8162)
  line L1006 (67.2702, 65.8162) -> (64.1702, 65.8162)
  line L1007 (64.1702, 65.8162) -> (64.1702, 74.4662)
  line L1008 (62.6702, 75.9662) -> (40.6452, 75.9662)
  line L1009 (40.6452, 75.9662) -> (40.6452, 53.9412)
  line L1010 (42.1452, 52.4412) -> (50.7952, 52.4412)
  line L1011 (50.7952, 52.4412) -> (50.7952, 49.3412)
  line L1012 (50.7952, 49.3412) -> (42.1452, 49.3412)
  line L1013 (40.6452, 47.8412) -> (40.6452, 25.8162)
  line L1014 (40.6452, 25.8162) -> (62.6702, 25.8162)
  line L1015 (64.1702, 27.3162) -> (64.1702, 35.9662)
  line L1016 (64.1702, 35.9662) -> (67.2702, 35.9662)
  line L1017 (67.2702, 35.9662) -> (67.2702, 27.3162)
  line L1018 (68.7702, 25.8162) -> (90.7952, 25.8162)
  line L1019 (90.7952, 25.8162) -> (90.7952, 47.8412)
  line L1020 (89.2952, 49.3412) -> (80.6452, 49.3412)
  line L1021 (80.6452, 49.3412) -> (80.6452, 52.4412)
  line L1022 (80.6452, 52.4412) -> (89.2952, 52.4412)
  line L1023 (90.7952, 53.9412) -> (90.7952, 75.9662)
  line L1024 (38.6452, 128.1161) -> (16.6202, 128.1161)
  line L1025 (15.1202, 126.6161) -> (15.1202, 117.9661)
  line L1026 (15.1202, 117.9661) -> (12.0202, 117.9661)
  line L1027 (12.0202, 117.9661) -> (12.0202, 126.6161)
  line L1028 (10.5202, 128.1161) -> (-11.5048, 128.1161)
  line L1029 (-11.5048, 128.1161) -> (-11.5048, 106.0911)
  line L1030 (-10.0048, 104.5911) -> (-1.3548, 104.5911)
  line L1031 (-1.3548, 104.5911) -> (-1.3548, 101.4911)
  line L1032 (-1.3548, 101.4911) -> (-10.0048, 101.4911)
  line L1033 (-11.5048, 99.9911) -> (-11.5048, 77.9661)
  line L1034 (-11.5048, 77.9661) -> (10.5202, 77.9661)
  line L1035 (12.0202, 79.4661) -> (12.0202, 88.1161)
  line L1036 (12.0202, 88.1161) -> (15.1202, 88.1161)
  line L1037 (15.1202, 88.1161) -> (15.1202, 79.4661)
  line L1038 (16.6202, 77.9661) -> (38.6452, 77.9661)
  line L1039 (38.6452, 77.9661) -> (38.6452, 99.9911)
  line L1040 (37.1452, 101.4911) -> (28.4952, 101.4911)
  line L1041 (28.4952, 101.4911) -> (28.4952, 104.5911)
  line L1042 (28.4952, 104.5911) -> (37.1452, 104.5911)
  line L1043 (38.6452, 106.0911) -> (38.6452, 128.1161)
  line L1044 (174.5594, 388.2371) -> (183.2094, 388.2371)
  line L1045 (184.7094, 389.7371) -> (184.7094, 399.2621)
  line L1046 (184.7094, 399.2621) -> (134.5594, 399.2621)
  line L1047 (134.5594, 399.2621) -> (134.5594, 389.7371)
  line L1048 (136.0594, 388.2371) -> (144.7094, 388.2371)
  line L1049 (144.7094, 388.2371) -> (144.7094, 385.1371)
  line L1050 (144.7094, 385.1371) -> (136.0594, 385.1371)
  line L1051 (134.5594, 383.6371) -> (134.5594, 374.1121)
  line L1052 (134.5594, 374.1121) -> (184.7094, 374.1121)
  line L1053 (184.7094, 374.1121) -> (184.7094, 383.6371)
  line L1054 (183.2094, 385.1371) -> (174.5594, 385.1371)
  line L1055 (174.5594, 385.1371) -> (174.5594, 388.2371)
  line L1056 (186.7093, 319.9621) -> (186.7093, 297.9371)
  line L1057 (188.2093, 296.4371) -> (196.8593, 296.4371)
  line L1058 (196.8593, 296.4371) -> (196.8593, 293.3371)
  line L1059 (196.8593, 293.3371) -> (188.2093, 293.3371)
  line L1060 (186.7093, 291.8371) -> (186.7093, 269.8121)
  line L1061 (186.7093, 269.8121) -> (208.7343, 269.8121)
  line L1062 (210.2343, 271.3121) -> (210.2343, 279.9621)
  line L1063 (210.2343, 279.9621) -> (213.3343, 279.9621)
  line L1064 (213.3343, 279.9621) -> (213.3343, 271.3121)
  line L1065 (214.8343, 269.8121) -> (236.8593, 269.8121)
  line L1066 (236.8593, 269.8121) -> (236.8593, 291.8371)
  line L1067 (235.3593, 293.3371) -> (226.7093, 293.3371)
  line L1068 (226.7093, 293.3371) -> (226.7093, 296.4371)
  line L1069 (226.7093, 296.4371) -> (235.3593, 296.4371)
  line L1070 (236.8593, 297.9371) -> (236.8593, 319.9621)
  line L1071 (236.8593, 319.9621) -> (214.8343, 319.9621)
  line L1072 (213.3343, 318.4621) -> (213.3343, 309.8121)
  line L1073 (213.3343, 309.8121) -> (210.2343, 309.8121)
  line L1074 (210.2343, 309.8121) -> (210.2343, 318.4621)
  line L1075 (208.7343, 319.9621) -> (186.7093, 319.9621)
  line L1076 (137.7525, 215.6625) -> (115.7275, 215.6625)
  line L1077 (114.2275, 214.1625) -> (114.2275, 205.5125)
  line L1078 (114.2275, 205.5125) -> (111.1275, 205.5125)
  line L1079 (111.1275, 205.5125) -> (111.1275, 214.1625)
  line L1080 (109.6275, 215.6625) -> (87.6025, 215.6625)
  line L1081 (87.6025, 215.6625) -> (87.6025, 193.6375)
  line L1082 (89.1025, 192.1375) -> (97.7525, 192.1375)
  line L1083 (97.7525, 192.1375) -> (97.7525, 189.0375)
  line L1084 (97.7525, 189.0375) -> (89.1025, 189.0375)
  line L1085 (87.6025, 187.5375) -> (87.6025, 165.5125)
  line L1086 (87.6025, 165.5125) -> (109.6275, 165.5125)
  line L1087 (111.1275, 167.0125) -> (111.1275, 175.6625)
  line L1088 (111.1275, 175.6625) -> (114.2275, 175.6625)
  line L1089 (114.2275, 175.6625) -> (114.2275, 167.0125)
  line L1090 (115.7275, 165.5125) -> (137.7525, 165.5125)
  line L1091 (137.7525, 165.5125) -> (137.7525, 187.5375)
  line L1092 (136.2525, 189.0375) -> (127.6025, 189.0375)
  line L1093 (127.6025, 189.0375) -> (127.6025, 192.1375)
  line L1094 (127.6025, 192.1375) -> (136.2525, 192.1375)
  line L1095 (137.7525, 193.6375) -> (137.7525, 215.6625)
  line L1096 (30.2591, 319.9624) -> (30.2591, 297.9374)
  line L1097 (31.7591, 296.4374) -> (40.4091, 296.4374)
  line L1098 (40.4091, 296.4374) -> (40.4091, 293.3374)
  line L1099 (40.4091, 293.3374) -> (31.7591, 293.3374)
  line L1100 (30.2591, 291.8374) -> (30.2591, 269.8124)
  line L1101 (30.2591, 269.8124) -> (52.2841, 269.8124)
  line L1102 (53.7841, 271.3124) -> (53.7841, 279.9624)
  line L1103 (53.7841, 279.9624) -> (56.8841, 279.9624)
  line L1104 (56.8841, 279.9624) -> (56.8841, 271.3124)
  line L1105 (58.3841, 269.8124) -> (80.4091, 269.8124)
  line L1106 (80.4091, 269.8124) -> (80.4091, 291.8374)
  line L1107 (78.9091, 293.3374) -> (70.2591, 293.3374)
  line L1108 (70.2591, 293.3374) -> (70.2591, 296.4374)
  line L1109 (70.2591, 296.4374) -> (78.9091, 296.4374)
  line L1110 (80.4091, 297.9374) -> (80.4091, 319.9624)
  line L1111 (80.4091, 319.9624) -> (58.3841, 319.9624)
  line L1112 (56.8841, 318.4624) -> (56.8841, 309.8124)
  line L1113 (56.8841, 309.8124) -> (53.7841, 309.8124)
  line L1114 (53.7841, 309.8124) -> (53.7841, 318.4624)
  line L1115 (52.2841, 319.9624) -> (30.2591, 319.9624)
  line L1116 (82.4091, 319.9624) -> (82.4091, 297.9374)
  line L1117 (83.9091, 296.4374) -> (92.5591, 296.4374)
  line L1118 (92.5591, 296.4374) -> (92.5591, 293.3374)
  line L1119 (92.5591, 293.3374) -> (83.9091, 293.3374)
  line L1120 (82.4091, 291.8374) -> (82.4091, 269.8124)
  line L1121 (82.4091, 269.8124) -> (104.4341, 269.8124)
  line L1122 (105.9341, 271.3124) -> (105.9341, 279.9624)
  line L1123 (105.9341, 279.9624) -> (109.0341, 279.9624)
  line L1124 (109.0341, 279.9624) -> (109.0341, 271.3124)
  line L1125 (110.5341, 269.8124) -> (132.5591, 269.8124)
  line L1126 (132.5591, 269.8124) -> (132.5591, 291.8374)
  line L1127 (131.0591, 293.3374) -> (122.4091, 293.3374)
  line L1128 (122.4091, 293.3374) -> (122.4091, 296.4374)
  line L1129 (122.4091, 296.4374) -> (131.0591, 296.4374)
  line L1130 (132.5591, 297.9374) -> (132.5591, 319.9624)
  line L1131 (132.5591, 319.9624) -> (110.5341, 319.9624)
  line L1132 (109.0341, 318.4624) -> (109.0341, 309.8124)
  line L1133 (109.0341, 309.8124) -> (105.9341, 309.8124)
  line L1134 (105.9341, 309.8124) -> (105.9341, 318.4624)
  line L1135 (104.4341, 319.9624) -> (82.4091, 319.9624)
  line L1136 (85.6027, 267.8124) -> (63.5777, 267.8124)
  line L1137 (62.0777, 266.3124) -> (62.0777, 257.6624)
  line L1138 (62.0777, 257.6624) -> (58.9777, 257.6624)
  line L1139 (58.9777, 257.6624) -> (58.9777, 266.3124)
  line L1140 (57.4777, 267.8124) -> (35.4527, 267.8124)
  line L1141 (35.4527, 267.8124) -> (35.4527, 245.7874)
  line L1142 (36.9527, 244.2874) -> (45.6027, 244.2874)
  line L1143 (45.6027, 244.2874) -> (45.6027, 241.1874)
  line L1144 (45.6027, 241.1874) -> (36.9527, 241.1874)
  line L1145 (35.4527, 239.6874) -> (35.4527, 217.6624)
  line L1146 (35.4527, 217.6624) -> (57.4777, 217.6624)
  line L1147 (58.9777, 219.1624) -> (58.9777, 227.8124)
  line L1148 (58.9777, 227.8124) -> (62.0777, 227.8124)
  line L1149 (62.0777, 227.8124) -> (62.0777, 219.1624)
  line L1150 (63.5777, 217.6624) -> (85.6027, 217.6624)
  line L1151 (85.6027, 217.6624) -> (85.6027, 239.6874)
  line L1152 (84.1027, 241.1874) -> (75.4527, 241.1874)
  line L1153 (75.4527, 241.1874) -> (75.4527, 244.2874)
  line L1154 (75.4527, 244.2874) -> (84.1027, 244.2874)
  line L1155 (85.6027, 245.7874) -> (85.6027, 267.8124)
  line L1156 (-11.5048, 75.9662) -> (-11.5048, 53.9412)
  line L1157 (-10.0048, 52.4412) -> (-1.3548, 52.4412)
  line L1158 (-1.3548, 52.4412) -> (-1.3548, 49.3412)
  line L1159 (-1.3548, 49.3412) -> (-10.0048, 49.3412)
  line L1160 (-11.5048, 47.8412) -> (-11.5048, 25.8162)
  line L1161 (-11.5048, 25.8162) -> (10.5202, 25.8162)
  line L1162 (12.0202, 27.3162) -> (12.0202, 35.9662)
  line L1163 (12.0202, 35.9662) -> (15.1202, 35.9662)
  line L1164 (15.1202, 35.9662) -> (15.1202, 27.3162)
  line L1165 (16.6202, 25.8162) -> (38.6452, 25.8162)
  line L1166 (38.6452, 25.8162) -> (38.6452, 47.8412)
  line L1167 (37.1452, 49.3412) -> (28.4952, 49.3412)
  line L1168 (28.4952, 49.3412) -> (28.4952, 52.4412)
  line L1169 (28.4952, 52.4412) -> (37.1452, 52.4412)
  line L1170 (38.6452, 53.9412) -> (38.6452, 75.9662)
  line L1171 (38.6452, 75.9662) -> (16.6202, 75.9662)
  line L1172 (15.1202, 74.4662) -> (15.1202, 65.8162)
  line L1173 (15.1202, 65.8162) -> (12.0202, 65.8162)
  line L1174 (12.0202, 65.8162) -> (12.0202, 74.4662)
  line L1175 (10.5202, 75.9662) -> (-11.5048, 75.9662)
  line L1176 (191.9024, 267.8121) -> (191.9024, 245.7871)
  line L1177 (193.4024, 244.2871) -> (202.0524, 244.2871)
  line L1178 (202.0524, 244.2871) -> (202.0524, 241.1871)
  line L1179 (202.0524, 241.1871) -> (193.4024, 241.1871)
  line L1180 (191.9024, 239.6871) -> (191.9024, 217.6621)
  line L1181 (191.9024, 217.6621) -> (213.9274, 217.6621)
  line L1182 (215.4274, 219.1621) -> (215.4274, 227.8121)
  line L1183 (215.4274, 227.8121) -> (218.5274, 227.8121)
  line L1184 (218.5274, 227.8121) -> (218.5274, 219.1621)
  line L1185 (220.0274, 217.6621) -> (242.0524, 217.6621)
  line L1186 (242.0524, 217.6621) -> (242.0524, 239.6871)
  line L1187 (240.5524, 241.1871) -> (231.9024, 241.1871)
  line L1188 (231.9024, 241.1871) -> (231.9024, 244.2871)
  line L1189 (231.9024, 244.2871) -> (240.5524, 244.2871)
  line L1190 (242.0524, 245.7871) -> (242.0524, 267.8121)
  line L1191 (242.0524, 267.8121) -> (220.0274, 267.8121)
  line L1192 (218.5274, 266.3121) -> (218.5274, 257.6621)
  line L1193 (218.5274, 257.6621) -> (215.4274, 257.6621)
  line L1194 (215.4274, 257.6621) -> (215.4274, 266.3121)
  line L1195 (213.9274, 267.8121) -> (191.9024, 267.8121)
  line L1196 (18.1092, 361.4411) -> (26.7592, 361.4411)
  line L1197 (28.2592, 362.9411) -> (28.2592, 372.4661)
  line L1198 (28.2592, 372.4661) -> (-21.8908, 372.4661)
  line L1199 (-21.8908, 372.4661) -> (-21.8908, 362.9411)
  line L1200 (-20.3908, 361.4411) -> (-11.7408, 361.4411)
  line L1201 (-11.7408, 361.4411) -> (-11.7408, 358.3411)
  line L1202 (-11.7408, 358.3411) -> (-20.3908, 358.3411)
  line L1203 (-21.8908, 356.8411) -> (-21.8908, 347.3161)
  line L1204 (-21.8908, 347.3161) -> (28.2592, 347.3161)
  line L1205 (28.2592, 347.3161) -> (28.2592, 356.8411)
  line L1206 (26.7592, 358.3411) -> (18.1092, 358.3411)
  line L1207 (18.1092, 358.3411) -> (18.1092, 361.4411)
  line L1208 (137.7527, 217.6624) -> (137.7527, 239.6874)
  line L1209 (136.2527, 241.1874) -> (127.6027, 241.1874)
  line L1210 (127.6027, 241.1874) -> (127.6027, 244.2874)
  line L1211 (127.6027, 244.2874) -> (136.2527, 244.2874)
  line L1212 (137.7527, 245.7874) -> (137.7527, 267.8124)
  line L1213 (137.7527, 267.8124) -> (115.7277, 267.8124)
  line L1214 (114.2277, 266.3124) -> (114.2277, 257.6624)
  line L1215 (114.2277, 257.6624) -> (111.1277, 257.6624)
  line L1216 (111.1277, 257.6624) -> (111.1277, 266.3124)
  line L1217 (109.6277, 267.8124) -> (87.6027, 267.8124)
  line L1218 (87.6027, 267.8124) -> (87.6027, 245.7874)
  line L1219 (89.1027, 244.2874) -> (97.7527, 244.2874)
  line L1220 (97.7527, 244.2874) -> (97.7527, 241.1874)
  line L1221 (97.7527, 241.1874) -> (89.1027, 241.1874)
  line L1222 (87.6027, 239.6874) -> (87.6027, 217.6624)
  line L1223 (87.6027, 217.6624) -> (109.6277, 217.6624)
  line L1224 (111.1277, 219.1624) -> (111.1277, 227.8124)
  line L1225 (111.1277, 227.8124) -> (114.2277, 227.8124)
  line L1226 (114.2277, 227.8124) -> (114.2277, 219.1624)
  line L1227 (115.7277, 217.6624) -> (137.7527, 217.6624)
  line L1228 (191.9024, 215.6621) -> (191.9024, 193.6371)
  line L1229 (193.4024, 192.1371) -> (202.0524, 192.1371)
  line L1230 (202.0524, 192.1371) -> (202.0524, 189.0371)
  line L1231 (202.0524, 189.0371) -> (193.4024, 189.0371)
  line L1232 (191.9024, 187.5371) -> (191.9024, 165.5121)
  line L1233 (191.9024, 165.5121) -> (213.9274, 165.5121)
  line L1234 (215.4274, 167.0121) -> (215.4274, 175.6621)
  line L1235 (215.4274, 175.6621) -> (218.5274, 175.6621)
  line L1236 (218.5274, 175.6621) -> (218.5274, 167.0121)
  line L1237 (220.0274, 165.5121) -> (242.0524, 165.5121)
  line L1238 (242.0524, 165.5121) -> (242.0524, 187.5371)
  line L1239 (240.5524, 189.0371) -> (231.9024, 189.0371)
  line L1240 (231.9024, 189.0371) -> (231.9024, 192.1371)
  line L1241 (231.9024, 192.1371) -> (240.5524, 192.1371)
  line L1242 (242.0524, 193.6371) -> (242.0524, 215.6621)
  line L1243 (242.0524, 215.6621) -> (220.0274, 215.6621)
  line L1244 (218.5274, 214.1621) -> (218.5274, 205.5121)
  line L1245 (218.5274, 205.5121) -> (215.4274, 205.5121)
  line L1246 (215.4274, 205.5121) -> (215.4274, 214.1621)
  line L1247 (213.9274, 215.6621) -> (191.9024, 215.6621)
  line L1248 (134.5592, 319.9623) -> (134.5592, 297.9373)
  line L1249 (136.0592, 296.4373) -> (144.7092, 296.4373)
  line L1250 (144.7092, 296.4373) -> (144.7092, 293.3373)
  line L1251 (144.7092, 293.3373) -> (136.0592, 293.3373)
  line L1252 (134.5592, 291.8373) -> (134.5592, 269.8123)
  line L1253 (134.5592, 269.8123) -> (156.5842, 269.8123)
  line L1254 (158.0842, 271.3123) -> (158.0842, 279.9623)
  line L1255 (158.0842, 279.9623) -> (161.1842, 279.9623)
  line L1256 (161.1842, 279.9623) -> (161.1842, 271.3123)
  line L1257 (162.6842, 269.8123) -> (184.7092, 269.8123)
  line L1258 (184.7092, 269.8123) -> (184.7092, 291.8373)
  line L1259 (183.2092, 293.3373) -> (174.5592, 293.3373)
  line L1260 (174.5592, 293.3373) -> (174.5592, 296.4373)
  line L1261 (174.5592, 296.4373) -> (183.2092, 296.4373)
  line L1262 (184.7092, 297.9373) -> (184.7092, 319.9623)
  line L1263 (184.7092, 319.9623) -> (162.6842, 319.9623)
  line L1264 (161.1842, 318.4623) -> (161.1842, 309.8123)
  line L1265 (161.1842, 309.8123) -> (158.0842, 309.8123)
  line L1266 (158.0842, 309.8123) -> (158.0842, 318.4623)
  line L1267 (156.5842, 319.9623) -> (134.5592, 319.9623)
  line L1268 (186.7093, 372.1121) -> (186.7093, 350.0871)
  line L1269 (188.2093, 348.5871) -> (196.8593, 348.5871)
  line L1270 (196.8593, 348.5871) -> (196.8593, 345.4871)
  line L1271 (196.8593, 345.4871) -> (188.2093, 345.4871)